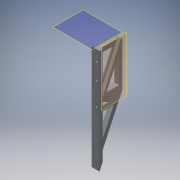
# Autodesk Inventor part: PlateSpacer
Saved by Autodesk Inventor 2016 (Build 200138000, 138)
## iProperties
Created: 2015-09-25
Part Number: PlateSpacer
Material: Generic
Document SubType Name: Modeling
Designer: Scott
Density: 1 g/cm^3
Appearance: Default
Author: Scott
Autodesk Inventor part; units mm, degrees
ref_plane "YZ Plane" through (0, 0, 0) normal (1, 0, 0) x (0, 1, 0)
ref_plane "XZ Plane" through (0, 0, 0) normal (0, 1, 0) x (-1, 0, 0)
ref_plane "Work Plane1" through (12.7, -42.953, -13.3823) normal (1, 0, 0) x (0, 1, 0)
sketch "Sketch1" plane through (12.7, -42.953, -13.3823) normal (1, 0, 0) x (0, 1, 0)
  line L0 (-54.71, 8.3023) -> (-54.71, 13.3823) projected
  line L1 (-54.71, 8.3023) -> (-47.0356, 8.3023) projected
  line L2 (-47.0356, 8.3023) -> (42.953, -31.0677) projected
  line L3 (42.953, -31.0677) -> (42.953, -10.5432) projected
  line L4 (42.953, -10.5432) -> (42.953, -7.1422) projected
  line L5 (42.953, -7.1422) -> (42.953, 13.3823) projected
  line L6 (42.953, 13.3823) -> (-54.71, 13.3823) projected
  line L7 (-18.8756, 8.3023) -> (29.7141, 8.3023) projected
  arc A0 (33.6511, 4.3653) -> (29.7141, 8.3023) centre (29.7141, 4.3653) ccw projected
  line L8 (33.6511, 4.3653) -> (33.6511, -16.8927) projected
  arc A1 (28.1361, -20.4997) -> (33.6511, -16.8927) centre (29.7141, -16.8927) ccw projected
  line L9 (28.1361, -20.4997) -> (-20.4536, 0.7583) projected
  arc A2 (-18.8756, 8.3023) -> (-20.4536, 0.7583) centre (-18.8756, 4.3653) ccw projected
  line L10 (-58.647, 13.3823) -> (-58.647, 8.3023) projected
  line L11 (-58.647, 13.3823) -> (-54.71, 13.3823) projected
  line L12 (-54.71, 8.3023) -> (-58.647, 8.3023) projected
  line L13 (42.953, 13.3823) -> (42.953, 19.7323)
  line L14 (42.953, 19.7323) -> (-160.247, 19.7323)
  line L15 (-160.247, 19.7323) -> (-50.8728, -31.0677)
  line L16 (-50.8728, -31.0677) -> (42.953, -31.0677)
  line L17 (42.953, -31.0677) -> (-47.0356, 8.3023)
  line L18 (-47.0356, 8.3023) -> (-47.0356, 0.7583)
  line L19 (-47.0356, 0.7583) -> (-58.647, 0.7583)
  line L20 (-58.647, 0.7583) -> (-58.647, 13.3823)
  line L21 (-58.647, 13.3823) -> (42.953, 13.3823)
  dimension "d0" = 6.35
  dimension "d1" = 203.2
  constraints: 18 end point, 4 perpendicular, 2 vertical, 1 collinear, 1 parallel
  measures "d0" distance of L5.end L13.end
  measures "d1" distance of L13.end L14.end
ref_plane "Work Plane2" through (0, -97.663, -42.3664) normal (-1, 0, 0) x (0, 0, 1)
extrude "Extrusion1" add sketch "Sketch1" against normal up to surface (12.7 mm away) contours L11 L10 L20 L19 L18 L2 L16 L15 L14 L13 L6
sketch "Sketch2" plane through (12.7, -203.2, 6.35) normal (0, 0, 1) x (1, 0, 0)
  circle A0 centre (-6.35, 182.88) radius 2.3495 projected
  circle A1 centre (-6.35, 151.13) radius 2.3495 projected
  circle A2 centre (-6.35, 106.68) radius 2.3495 projected
  point P0 (-12.7, 203.2)
extrude "Extrusion2" cut sketch "Sketch2" against normal blind 17.4625
sketch "Sketch3" plane through (0, -203.2, 6.35) normal (-1, 0, 0) x (0, 0, 1)
  line L0 (0, 203.2) -> (0, 0) projected
  line L1 (-6.35, 203.2) -> (0, 203.2) projected
  line L2 (-6.35, 101.6) -> (-6.35, 203.2) projected
  line L3 (-18.9739, 101.6) -> (-6.35, 101.6) projected
  line L4 (-18.9739, 113.2114) -> (-18.9739, 101.6) projected
  line L5 (-11.43, 113.2114) -> (-18.9739, 113.2114) projected
  line L6 (-50.8, 203.2) -> (-11.43, 113.2114) projected
  line L7 (-50.8, 109.3742) -> (-50.8, 203.2) projected
  line L8 (0, 0) -> (-50.8, 109.3742) projected
  line L9 (-35.8, 198.4375) -> (-35.8, 203.2) projected
  line L10 (-15.367, 193.8982) -> (-36.625, 193.8982) projected
  line L11 (0, 109.0295) -> (0, 104.3305) projected
  line L12 (-50.8, 193.8982) -> (0, 193.8982)
  line L13 (0, 193.8982) -> (0, 109.0295)
  line L14 (0, 109.0295) -> (-50.8, 109.0295)
  line L15 (-50.8, 109.0295) -> (-50.8, 193.8982)
  constraints: 8 end point, 2 parallel, 1 horizontal, 1 perpendicular, 1 point on line
extrude "Extrusion3" add sketch "Sketch3" along normal blind 2.54 contours L0 L12 L2 L1 | L0 L14 L2 L12 | L0 L8 L14 L4 L3 L2 | L2 L14 L4 L5 L6 L12 L10 | L14 L8 L7 L12 L6 L5 L4 | L14 L15 L8 | L12 L7 L6
sketch "Sketch4" plane through (0, -203.2, 6.35) normal (1, 0, 0) x (0, 0, -1)
  line L0 (11.43, 141.3714) -> (11.43, 189.9612) projected
  line L1 (11.43, 105.537) -> (6.35, 105.537) projected
  line L2 (11.43, 105.537) -> (11.43, 113.2114) projected
  line L3 (11.43, 113.2114) -> (50.8, 203.2) projected
  line L4 (50.8, 203.2) -> (30.2755, 203.2) projected
  line L5 (30.2755, 203.2) -> (26.8745, 203.2) projected
  line L6 (26.8745, 203.2) -> (6.35, 203.2) projected
  line L7 (6.35, 203.2) -> (6.35, 105.537) projected
  line L8 (11.43, 141.3714) -> (11.43, 189.9612) projected
  arc A0 (15.367, 193.8982) -> (11.43, 189.9612) centre (15.367, 189.9612) ccw projected
  line L9 (15.367, 193.8982) -> (36.625, 193.8982) projected
  arc A1 (40.2319, 188.3831) -> (36.625, 193.8982) centre (36.625, 189.9612) ccw projected
  line L10 (40.2319, 188.3831) -> (18.9739, 139.7934) projected
  arc A2 (11.43, 141.3714) -> (18.9739, 139.7934) centre (15.367, 141.3714) ccw projected
  line L11 (11.43, 185.3087) -> (38.8868, 185.3087)
  constraints: 2 end point, 2 point on line, 1 perpendicular
extrude "Extrusion4" cut sketch "Sketch4" against normal blind 2.54 contours L0 L11 L10 A2
fillet "Fillet1" radius 3.175 1 edges at (6.35, -89.9886, -5.08)
fillet "Fillet2" radius 1.5875 1 edges at (5.08, 0, -44.45)
sketch "Sketch5" plane through (12.7, -42.953, -13.3823) normal (1, 0, 0) x (0, 0, -1)
  arc A0 (31.0677, 35.3637) -> (28.0258, 36) centre (29.4802, 35.3637) ccw projected
  line L0 (28.0258, 36) -> (-6.3564, -42.588) projected
  arc A1 (-6.3564, -42.588) -> (-3.4476, -47.0356) centre (-3.4476, -43.8606) ccw projected
  line L1 (-3.4476, -47.0356) -> (-0.7583, -47.0356) projected
  line L2 (-0.7583, -47.0356) -> (-0.7583, -58.647) projected
  line L3 (-0.7583, -58.647) -> (-13.3823, -58.647) projected
  line L4 (-13.3823, -58.647) -> (-13.3823, 42.953) projected
  line L5 (-13.3823, 42.953) -> (-19.7323, 42.953) projected
  line L6 (-19.7323, 42.953) -> (-19.7323, -160.247) projected
  line L7 (-19.7323, -160.247) -> (31.0677, -50.8728) projected
  line L8 (31.0677, -50.8728) -> (31.0677, 35.3637) projected
  line L9 (-13.3823, -127.1164) -> (-13.3823, -67.9876)
  line L10 (-13.3823, -127.1164) -> (14.3959, -67.9876)
  line L11 (14.3959, -67.9876) -> (-13.3823, -67.9876)
  line L12 (2.8311, -39.9014) -> (24.5341, -39.9014)
  line L13 (24.5341, -39.9014) -> (24.5341, 13.7178)
  line L14 (24.5341, 13.7178) -> (0.5068, -39.9014)
  line L15 (0.5068, -39.9014) -> (2.8311, -39.9014)
  constraints: 14 end point, 2 horizontal, 1 collinear, 1 parallel, 1 vertical
extrude "Extrusion5" cut sketch "Sketch5" against normal blind 17.78 contours L9 L11 L10 | L15 L14 L13 L12
chamfer "Chamfer1" distance 12.7 angle 45 1 edges at (12.7, -95.7943, -12.6239)
ref_plane "Work Plane3" through (6.35, 0, 0) normal (0, -1, 0) x (1, 0, 0)
sketch "Sketch6" plane through (12.7, -110.9406, -27.7782) normal (0, -1, 0) x (1, 0, 0)
  line L0 (-15.24, 34.1282) -> (-15.24, 27.7782) projected
  line L1 (-15.24, 34.1282) -> (-15.24, 27.7782)
  line L2 (0, 27.7782) -> (0, 0) projected
  line L3 (0, -16.6718) -> (-12.7, -16.6718) projected
  line L4 (0, 27.7782) -> (-6.35, 27.7782)
  line L5 (-6.35, 27.7782) -> (-6.35, -16.6718)
  line L6 (-6.35, -16.6718) -> (0, -16.6718)
  line L7 (0, -16.6718) -> (0, 27.7782)
  point P0 (-12.7, 27.7782)
  dimension "d17" = 6.35
  dimension "d18" = 6.35
  constraints: 10 end point, 2 parallel, 1 horizontal, 1 midpoint, 1 perpendicular, 1 point on line
  measures "d17" distance of L0.start L1.end
  measures "d18" distance of L6.end L5.end
extrude "Extrusion6" cut sketch "Sketch6" along normal mid plane 211.455
body "Solid1"
